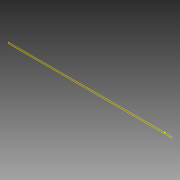
# Autodesk Inventor part: Panel_front
Saved by Autodesk Inventor 2013 (Build 170138000, 138)
## iProperties
Created: 2013-02-01
Part Number: Panel_front
Material: Aluminum 6061
Document SubType Name: Modeling
Designer: xylzlyx
Density: 1 g/cm^3
Author: xylzlyx
Autodesk Inventor part; units mm, degrees
ref_plane "YZ Plane" through (0, 0, 0) normal (1, 0, 0) x (0, 1, 0)
ref_plane "XZ Plane" through (0, 0, 0) normal (0, 1, 0) x (-1, 0, 0)
ref_plane "XY Plane" through (0, 0, 0) normal (0, 0, 1) x (1, 0, 0)
ref_plane "RecessedFrontPanel" through (0, 0, -4) normal (0, 0, 1) x (1, 0, 0)
sketch "Sketch2" plane through (0, 0, -4) normal (0, 0, 1) x (1, 0, 0)
  line L0 (0, -3) -> (-375, -3) construction
  line L1 (-375, -3) -> (-375, 0) construction
  line L2 (-375, 0) -> (0, 0) construction
  line L3 (0, 0) -> (0, -3) construction
  line L4 (-375, 55.1856) -> (-375, 58.2318) construction
  line L5 (-375, 58.2318) -> (0, 58.2318) construction
  line L6 (0, 58.2318) -> (0, 55.1856) construction
  line L7 (0, 55.1856) -> (-375, 55.1856) construction
  line L8 (-375, 54.6856) -> (0, 54.6856)
  line L9 (0, 54.6856) -> (0, 0)
  line L10 (0, 0) -> (-375, 0)
  line L11 (-375, 0) -> (-375, 54.6856)
  dimension "d1" = 0.5
  constraints: 24 end point, 5 horizontal, 4 vertical, 2 parallel, 2 vertical alignment, 1 coincident, 1 perpendicular, 7 other
  measures "d1" distance between parallel lines of L7 L8
extrude "Extrusion1" add sketch "Sketch2" against normal blind 3
fillet "Fillet1" radius 1 4 edges at (-375, 54.6856, -5.5) (-375, 0, -5.5) (0, 0, -5.5) (0, 54.6856, -5.5)
body "Solid1"
